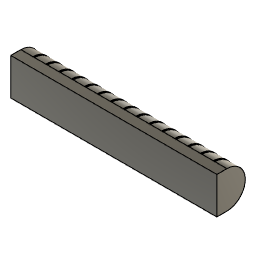
Front Greeblie LG (Autodesk Fusion 360 design; units mm, degrees)
Autodesk Fusion 360 part; units mm, degrees
sketch "Sketch1" plane through (0, 0, 0) normal (1, 0, 0) x (0, 1, 0)
  circle A0 centre (0, 0) radius 2.75
  line L0 (0, 0) -> (0, 2.75) construction
  line L1 (0, 0) -> (0, -2.75) construction
  line L2 (0, 2.75) -> (-1.5, 2.75)
  line L3 (-1.5, 2.75) -> (-1.5, -2.75)
  line L4 (-1.5, -2.75) -> (0, -2.75)
  line L5 (0, -2.75) -> (0, 2.75)
  dimension "d1" = 5.5
  dimension "d79" = 1.5
  constraint coincident A0.centre L0.start
  constraint coincident A0 L0.end
  constraint vertical L0
  constraint coincident A0 L1.end
  constraint parallel L0 L1
  constraint horizontal L2
  constraint vertical L3
  constraint horizontal L4
  constraint vertical L5
  measures "d1" diameter of A0
  measures "d79" distance of L0.end L2.end
extrude "Extrude1" add sketch "Sketch1" along normal mid plane 30.8 contours A0 L5 | A0 L3 L5 | A0 L3
ref_plane "WorkPlane1" through (0, 0, 0) normal (1, 0, 0) x (0, 1, 0)
sketch "Sketch2" plane through (0, 0, 0) normal (1, 0, 0) x (0, 1, 0)
  circle A0 centre (0, 0) radius 2.75
  circle A1 centre (0, 0) radius 2.625
  dimension "d5" = 5.5
  dimension "d6" = 5.25
  constraint coincident A0.centre A1.centre
  measures "d5" diameter of A0
  measures "d6" diameter of A1
extrude "Extrude2" cut sketch "Sketch2" along normal mid plane 0.25
ref_plane "WorkPlane2" through (7.7, 0, 0) normal (1, 0, 0) x (0, 1, 0)
sketch "Sketch3" plane through (7.7, 0, 0) normal (1, 0, 0) x (0, 1, 0)
  circle A0 centre (0, 0) radius 2.75
  circle A1 centre (0, 0) radius 2.625
  dimension "d10" = 5.5
  dimension "d11" = 5.25
  constraint coincident A0.centre A1.centre
  constraint concentric A0 A1
  measures "d10" diameter of A0
  measures "d11" diameter of A1
extrude "Extrude3" cut sketch "Sketch3" along normal mid plane 0.25
ref_plane "WorkPlane3" through (11.55, 0, 0) normal (1, 0, 0) x (0, 1, 0)
sketch "Sketch4" plane through (11.55, 0, 0) normal (1, 0, 0) x (0, 1, 0)
  circle A0 centre (0, 0) radius 2.75
  circle A1 centre (0, 0) radius 2.625
  dimension "d15" = 5.5
  dimension "d16" = 5.25
  constraint coincident A0.centre A1.centre
  constraint concentric A0 A1
  measures "d15" diameter of A0
  measures "d16" diameter of A1
extrude "Extrude4" cut sketch "Sketch4" along normal mid plane 0.25
ref_plane "WorkPlane4" through (13.475, 0, 0) normal (1, 0, 0) x (0, 1, 0)
sketch "Sketch5" plane through (13.475, 0, 0) normal (1, 0, 0) x (0, 1, 0)
  circle A0 centre (0, 0) radius 2.75
  circle A1 centre (0, 0) radius 2.625
  dimension "d20" = 5.5
  dimension "d21" = 5.25
  constraint coincident A0.centre A1.centre
  constraint concentric A0 A1
  measures "d20" diameter of A0
  measures "d21" diameter of A1
extrude "Extrude5" cut sketch "Sketch5" along normal mid plane 0.25
ref_plane "WorkPlane5" through (9.625, 0, 0) normal (1, 0, 0) x (0, 1, 0)
sketch "Sketch6" plane through (9.625, 0, 0) normal (1, 0, 0) x (0, 1, 0)
  circle A0 centre (0, 0) radius 2.75
  circle A1 centre (0, 0) radius 2.625
  dimension "d25" = 5.5
  dimension "d26" = 5.25
  constraint coincident A0.centre A1.centre
  constraint concentric A0 A1
  measures "d25" diameter of A0
  measures "d26" diameter of A1
extrude "Extrude6" cut sketch "Sketch6" along normal mid plane 0.25
ref_plane "WorkPlane6" through (5.775, 0, 0) normal (1, 0, 0) x (0, 1, 0)
sketch "Sketch7" plane through (5.775, 0, 0) normal (1, 0, 0) x (0, 1, 0)
  circle A0 centre (0, 0) radius 2.75
  circle A1 centre (0, 0) radius 2.625
  dimension "d30" = 5.5
  dimension "d31" = 5.25
  constraint coincident A0.centre A1.centre
  measures "d30" diameter of A0
  measures "d31" diameter of A1
extrude "Extrude7" cut sketch "Sketch7" along normal mid plane 0.25
ref_plane "WorkPlane7" through (3.85, 0, 0) normal (1, 0, 0) x (0, 1, 0)
sketch "Sketch8" plane through (3.85, 0, 0) normal (1, 0, 0) x (0, 1, 0)
  circle A0 centre (0, 0) radius 2.75
  circle A1 centre (0, 0) radius 2.625
  dimension "d35" = 5.5
  dimension "d36" = 5.25
  constraint coincident A0.centre A1.centre
  measures "d35" diameter of A0
  measures "d36" diameter of A1
extrude "Extrude8" cut sketch "Sketch8" along normal mid plane 0.25
ref_plane "WorkPlane8" through (1.925, 0, 0) normal (1, 0, 0) x (0, 1, 0)
sketch "Sketch9" plane through (1.925, 0, 0) normal (1, 0, 0) x (0, 1, 0)
  circle A0 centre (0, 0) radius 2.75
  circle A1 centre (0, 0) radius 2.625
  dimension "d40" = 5.5
  dimension "d41" = 5.25
  constraint coincident A0.centre A1.centre
  measures "d40" diameter of A0
  measures "d41" diameter of A1
extrude "Extrude9" cut sketch "Sketch9" along normal mid plane 0.25
ref_plane "WorkPlane9" through (-13.475, 0, 0) normal (-1, 0, 0) x (0, -1, 0)
sketch "Sketch10" plane through (-13.475, 0, 0) normal (-1, 0, 0) x (0, 1, 0)
  circle A0 centre (0, 0) radius 2.75
  circle A1 centre (0, 0) radius 2.625
  dimension "d45" = 5.5
  dimension "d46" = 5.25
  constraint coincident A0.centre A1.centre
  constraint concentric A0 A1
  measures "d45" diameter of A0
  measures "d46" diameter of A1
extrude "Extrude10" cut sketch "Sketch10" along normal mid plane 0.25
ref_plane "WorkPlane10" through (-11.55, 0, 0) normal (-1, 0, 0) x (0, -1, 0)
sketch "Sketch11" plane through (-11.55, 0, 0) normal (-1, 0, 0) x (0, 1, 0)
  circle A0 centre (0, 0) radius 2.75
  circle A1 centre (0, 0) radius 2.625
  dimension "d50" = 5.5
  dimension "d51" = 5.25
  constraint coincident A0.centre A1.centre
  measures "d50" diameter of A0
  measures "d51" diameter of A1
extrude "Extrude11" cut sketch "Sketch11" along normal mid plane 0.25
ref_plane "WorkPlane11" through (-9.625, 0, 0) normal (-1, 0, 0) x (0, -1, 0)
sketch "Sketch12" plane through (-9.625, 0, 0) normal (-1, 0, 0) x (0, 1, 0)
  circle A0 centre (0, 0) radius 2.75
  circle A1 centre (0, 0) radius 2.625
  dimension "d55" = 5.5
  dimension "d56" = 5.25
  constraint coincident A0.centre A1.centre
  constraint concentric A0 A1
  measures "d55" diameter of A0
  measures "d56" diameter of A1
extrude "Extrude12" cut sketch "Sketch12" along normal mid plane 0.25
ref_plane "WorkPlane12" through (-7.7, 0, 0) normal (-1, 0, 0) x (0, -1, 0)
sketch "Sketch13" plane through (-7.7, 0, 0) normal (-1, 0, 0) x (0, 1, 0)
  circle A0 centre (0, 0) radius 2.75
  circle A1 centre (0, 0) radius 2.625
  dimension "d60" = 5.5
  dimension "d61" = 5.25
  constraint coincident A0.centre A1.centre
  measures "d60" diameter of A0
  measures "d61" diameter of A1
extrude "Extrude13" cut sketch "Sketch13" along normal mid plane 0.25
ref_plane "WorkPlane13" through (-5.775, 0, 0) normal (-1, 0, 0) x (0, -1, 0)
sketch "Sketch14" plane through (-5.775, 0, 0) normal (-1, 0, 0) x (0, 1, 0)
  circle A0 centre (0, 0) radius 2.75
  circle A1 centre (0, 0) radius 2.625
  dimension "d65" = 5.5
  dimension "d66" = 5.25
  constraint coincident A0.centre A1.centre
  constraint concentric A0 A1
  measures "d65" diameter of A0
  measures "d66" diameter of A1
extrude "Extrude14" cut sketch "Sketch14" along normal mid plane 0.25
ref_plane "WorkPlane14" through (-3.85, 0, 0) normal (-1, 0, 0) x (0, -1, 0)
sketch "Sketch15" plane through (-3.85, 0, 0) normal (-1, 0, 0) x (0, 1, 0)
  circle A0 centre (0, 0) radius 2.75
  circle A1 centre (0, 0) radius 2.625
  dimension "d70" = 5.5
  dimension "d71" = 5.25
  constraint coincident A0.centre A1.centre
  measures "d70" diameter of A0
  measures "d71" diameter of A1
extrude "Extrude15" cut sketch "Sketch15" along normal mid plane 0.25
ref_plane "WorkPlane15" through (-1.925, 0, 0) normal (-1, 0, 0) x (0, -1, 0)
sketch "Sketch16" plane through (-1.925, 0, 0) normal (-1, 0, 0) x (0, 1, 0)
  circle A0 centre (0, 0) radius 2.75
  circle A1 centre (0, 0) radius 2.625
  dimension "d75" = 5.5
  dimension "d76" = 5.25
  constraint coincident A0.centre A1.centre
  measures "d75" diameter of A0
  measures "d76" diameter of A1
extrude "Extrude16" cut sketch "Sketch16" along normal mid plane 0.25
extrude "Extrude17" add sketch "Sketch1" along normal mid plane 30.8 contours A0 L3 L5 | A0 L2 L3 | A0 L3 L4
extrude "Extrude18" cut sketch "Sketch1" along normal mid plane 30.8 contours A0 L3
